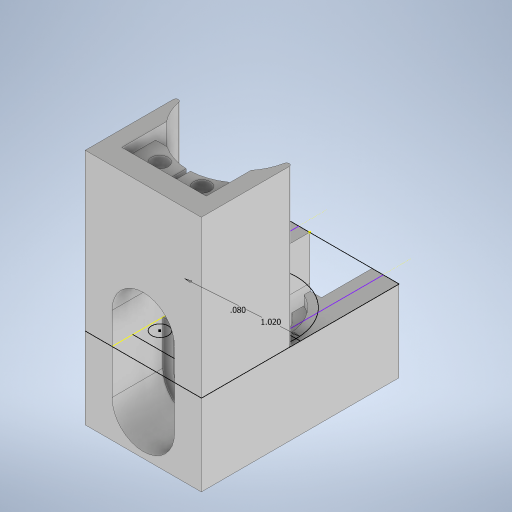
# Autodesk Inventor part: Ball Valve Mount 2
Saved by Autodesk Inventor 2024 (Build 280153000, 153)
## iProperties
Created: 2023-02-08
Part Number: Ball Valve Mount 2
Material: Generic
Document SubType Name: Modeling
Designer: tommy
Density: 1 g/cm^3
Appearance: Default
Author: tommy
Autodesk Inventor part; units mm, degrees
ref_plane "YZ Plane" through (0, 0, 0) normal (1, 0, 0) x (0, 1, 0)
ref_plane "XZ Plane" through (0, 0, 0) normal (0, 1, 0) x (-1, 0, 0)
ref_plane "XY Plane" through (0, 0, 0) normal (0, 0, 1) x (1, 0, 0)
sketch "Sketch1" plane through (0, 0, 0) normal (0, 1, 0) x (-1, 0, 0)
  circle A0 centre (0, 0) radius 8.636
  line L0 (7.5565, 23.7871) -> (-7.5565, 23.7871)
  line L1 (7.5565, -23.7871) -> (-7.5565, -23.7871)
  line L2 (7.5565, 23.7871) -> (7.5565, 8.2342)
  line L3 (7.5565, -8.2342) -> (7.5565, -23.7871)
  arc A1 (7.5565, -8.2342) -> (7.5565, 8.2342) centre (0, 0) ccw
  arc A2 (-7.5565, 8.2342) -> (-7.5565, -8.2342) centre (0, 0) ccw
  line L4 (-7.5565, -23.7871) -> (-7.5565, -8.2342)
  line L5 (-7.5565, 8.2342) -> (-7.5565, 23.7871)
  line L6 (-9.144, -8.9047) -> (-9.144, -23.7871)
  line L7 (9.144, -23.7871) -> (9.144, -8.9047)
  arc A3 (9.144, -8.9047) -> (9.144, 8.9047) centre (0, 0) ccw
  line L8 (9.144, 8.9047) -> (9.144, 23.7871)
  line L9 (-9.144, 23.7871) -> (-9.144, 8.9047)
  arc A4 (-9.144, 8.9047) -> (-9.144, -8.9047) centre (0, 0) ccw
  line L10 (7.5565, -23.7871) -> (9.144, -23.7871)
  line L11 (9.144, -23.7871) -> (-9.144, -23.7871)
  line L12 (-7.5565, 23.7871) -> (-9.144, 23.7871)
  line L13 (-9.144, 23.7871) -> (9.144, 23.7871)
  circle A5 centre (0, 0) radius 11.176
  line L14 (46.1577, 0) -> (-42.2099, 0)
  circle A6 centre (-19.5645, 19.9771) radius 2.0193
  circle A7 centre (0, 0) radius 2.921 construction
  circle A8 centre (0, 0) radius 6.604 construction
  line L15 (-6.3706, -6.3706) -> (-16.823, -4.7025) construction
  arc A9 (0, 23.3745) -> (-23.2624, -2.286) centre (0, 0) ccw construction
  line L16 (4.7025, 16.823) -> (6.3706, 6.3706) construction
  arc A10 (-20.8345, 0) -> (-16.823, -4.7025) centre (-16.0725, 0) ccw construction
  line L17 (-4.7025, -16.823) -> (-6.3706, -6.3706) construction
  arc A11 (-4.7025, -16.823) -> (0, -20.8345) centre (0, -16.0725) ccw construction
  arc A12 (4.7025, 16.823) -> (0, 20.8345) centre (0, 16.0725) ccw construction
  line L18 (6.3706, 6.3706) -> (16.823, 4.7025) construction
  arc A13 (20.8345, 0) -> (16.823, 4.7025) centre (16.0725, 0) ccw construction
  arc A14 (0, -20.8345) -> (20.8345, 0) centre (0, 0) ccw construction
  line L19 (2.286, -2.286) -> (-23.2624, -2.286) construction
  line L20 (-10.16, 30.48) -> (10.16, 30.48) construction
  circle A15 centre (-5.08, 34.544) radius 2.0193 construction
  line L21 (-13.97, 38.608) -> (13.97, 38.608) construction
  circle A16 centre (5.08, 34.544) radius 2.0193 construction
  line L22 (-0.508, 30.48) -> (-0.508, 38.608) construction
  line L23 (0.508, 30.48) -> (0.508, 38.608) construction
  line L24 (-10.16, -10.668) -> (-10.16, 30.48) construction
  line L25 (10.16, 9.906) -> (-10.16, 9.906) construction
  line L26 (13.97, 38.608) -> (13.97, -18.796) construction
  line L27 (-13.97, -18.796) -> (-13.97, 38.608) construction
  line L28 (10.16, 30.48) -> (10.16, -10.668) construction
  circle A17 centre (0, 0) radius 6.604 construction
  line L29 (10.16, -10.668) -> (-10.16, -10.668) construction
  circle A18 centre (5.08, -14.732) radius 2.0193 construction
  circle A19 centre (-5.08, -14.732) radius 2.0193 construction
  line L30 (-0.508, -18.796) -> (-0.508, -10.668) construction
  line L31 (0.508, -18.796) -> (0.508, -10.668) construction
  line L32 (-4.7025, -16.823) -> (-4.7191, -16.7188) construction
  line L33 (-4.7025, -16.823) -> (-4.7191, -16.7188) construction
  line L34 (13.97, -18.796) -> (-13.97, -18.796) construction
  arc A20 (0, 20.8345) -> (-20.8345, 0) centre (0, 0) ccw construction
  line L35 (0, 0) -> (0, 23.3745) construction
  line L36 (-23.3745, 0) -> (-23.3745, 23.7871)
  line L37 (-23.3745, 23.7871) -> (-9.144, 23.7871)
  line L38 (20.8345, 0) -> (20.8345, 23.7871)
  line L39 (20.8345, 23.7871) -> (9.144, 23.7871)
  line L40 (-23.3745, 0) -> (-23.3745, -18.796)
  line L41 (20.8345, 0) -> (20.8345, -18.796)
  arc A21 (-7.5565, 22.5203) -> (-23.3745, 4.2308) centre (0, 0) ccw
  arc A22 (7.5565, -19.8241) -> (20.8345, -4.0026) centre (0, 0) ccw
  arc A23 (20.8345, 1.9426) -> (17.0954, 5.0402) centre (16.0725, 0) ccw
  line L42 (17.0954, 5.0402) -> (11.748, 5.8959)
  circle A24 centre (0, 0) radius 12.7635 construction
  arc A25 (-20.4699, -2.667) -> (-16.883, -5.0787) centre (-16.0725, 0) ccw
  line L43 (-16.883, -5.0787) -> (-11.7468, -5.8984)
  line L44 (-20.4699, -2.667) -> (-23.3745, -2.667)
  arc A26 (-11.7468, -5.8984) -> (-7.5565, -10.7553) centre (0, 0) ccw
  arc A27 (11.748, 5.8959) -> (7.5565, 10.7553) centre (0, 0) ccw
  circle A28 centre (17.0245, 19.9771) radius 2.0193
  circle A29 centre (17.0245, -19.9771) radius 2.0193
  circle A30 centre (-17.0245, -17.4371) radius 2.0193
  line L45 (-9.144, -18.796) -> (-7.5565, -18.796)
  circle A31 centre (-19.5645, 19.9771) radius 2.286
  circle A32 centre (-17.0245, -17.4371) radius 2.286
  circle A33 centre (17.0245, -19.9771) radius 2.286
  circle A34 centre (17.0245, 19.9771) radius 2.286
  arc A35 (-9.144, 8.9047) -> (-9.144, -8.9047) centre (0, 0) ccw
  line L46 (-9.144, -8.9047) -> (-9.144, -18.796)
  line L47 (-23.3745, -18.796) -> (-23.3745, 23.7871)
  line L48 (-23.3745, 23.7871) -> (-9.144, 23.7871)
  line L49 (-9.144, 23.7871) -> (-9.144, 8.9047)
  line L50 (20.8345, -18.796) -> (20.8345, 23.7871)
  line L51 (20.8345, 23.7871) -> (9.144, 23.7871)
  line L52 (9.144, 23.7871) -> (9.144, 8.9047)
  line L53 (9.144, -18.796) -> (9.144, -8.9047)
  arc A36 (9.144, -8.9047) -> (9.144, 8.9047) centre (0, 0) ccw
  line L54 (9.144, -23.7871) -> (20.8345, -23.7871)
  line L55 (20.8345, -23.7871) -> (20.8345, -18.796)
  line L56 (-9.144, -23.7871) -> (-23.3745, -23.7871)
  line L57 (-23.3745, -23.7871) -> (-23.3745, -18.796)
  point P0 (-7.5565, -8.2342)
  point P1 (-7.5565, 8.2342)
  point P2 (-12.7635, 0)
  point P3 (-8.636, 0)
  point P4 (8.636, 0)
  point P5 (12.7635, 0)
  point P6 (-12.7635, 0)
  point P7 (0, 9.906)
  point P8 (-9.144, 21.9238)
  point P9 (9.8391, -18.796)
  point P10 (9.144, -19.1438)
  point P11 (-9.144, -9.4427)
  point P12 (-9.144, -9.4427)
  dimension "d12" = 18.161
  dimension "d0" = 17.272
  dimension "d6" = 15.113
  dimension "d7" = 1.5875
  dimension "d27" = 4.0386
  dimension "d31" = 5.842
  dimension "d32" = 13.208
  dimension "d38" = 41.148
  dimension "d39" = 20.32
  dimension "d40" = 4.0386
  dimension "d41" = 4.0386
  dimension "d49" = 13.208
  dimension "d55" = 3.81
  dimension "d56" = 3.81
  dimension "d57" = 19.5645
  dimension "d59" = 4.0386
  dimension "d60" = 4.0386
  dimension "d61" = 4.0386
  dimension "d62" = 3.81
  dimension "d64" = 6.35
  dimension "d66" = 3.81
  dimension "d67" = 3.81
  dimension "d68" = 4.572
  dimension "d69" = 4.572
  dimension "d70" = 4.572
  dimension "d71" = 4.572
  dimension "d90" = 3.81
  dimension "d91" = 6.35
  constraints: 114 end point, 44 point on circle, 35 centre point, 24 point on line, 16 perpendicular, 10 coincident, 5 parallel, 5 tangent, 4 horizontal, 4 vertical, 3 midpoint, 2 collinear, 1 concentric, 1 horizontal alignment, 15 other
  measures "d0" diameter of A0
  measures "d6" distance of L0.start L0.end
  measures "d7" distance between parallel lines of L4 L6
  measures "d27" diameter of A6
  measures "d31" diameter of A7
  measures "d32" diameter of A8
  measures "d38" distance of L28.start L28.end
  measures "d39" distance of L24.end L28.start
  measures "d40" diameter of A16
  measures "d41" diameter of A18
  measures "d49" diameter of A17
  measures "d55" distance from line of L36 A6.centre
  measures "d56" distance from line of L37 A6.centre
  measures "d57" distance from line of L35 A6.centre
  measures "d59" diameter of A28
  measures "d60" diameter of A29
  measures "d61" diameter of A30
  measures "d62" distance from line of L41 A29.centre
  measures "d64" distance from line of L40 A30.centre
  measures "d66" distance from line of L38 A28.centre
  measures "d67" distance from line of L39 A28.centre
  measures "d68" diameter of A31
  measures "d69" diameter of A32
  measures "d70" diameter of A33
  measures "d71" diameter of A34
  measures "d90" distance from line of L54 A29.centre
  measures "d91" distance from line of L56 A30.centre
extrude "Extrusion1" add sketch "Sketch1" along normal blind 18.796 contours A0 L14 A2 A5 A1 | A1 L2 A27 L8 A3 L14 | L14 A4 L9 A21 L5 A2 | A5 L5 L0 L2 | L2 L13 L8 A27 | A21 L9 L12 L5 picked at (-5.9238, 8.392)
extrude "Extrusion2" cut sketch "Sketch1" along normal blind 2.286 contours L14 A1 A5 A2 A0 | A0 L14 A2 A5 A1
sketch "Sketch2" plane through (-9.144, 0, 23.7871) normal (0, 0, 1) x (1, 0, 0)
  line L0 (9.144, 0) -> (9.144, 18.161)
  line L1 (9.144, 18.161) -> (9.144, 10.6426)
  circle A0 centre (9.144, 10.6426) radius 7.5184
  line L2 (16.6624, 10.6426) -> (16.6624, -7.5184)
  line L3 (20.32, 0) -> (-2.032, 0) projected
  line L4 (1.6256, 10.6426) -> (1.6256, -7.5184)
  line L5 (1.6256, 0) -> (16.6624, 0)
  circle A1 centre (9.144, 10.6426) radius 4.826
  line L6 (4.318, 10.6426) -> (4.318, 0)
  line L7 (13.97, 10.6426) -> (13.97, 0)
  line L8 (18.288, 0) -> (0, 0) projected
  circle A2 centre (9.144, -7.5184) radius 7.5184
  line L9 (1.6256, 10.6426) -> (16.6624, 10.6426)
  point P0 (4.318, 0)
  point P1 (4.318, 5.7651)
  point P2 (13.97, 5.7651)
  point P3 (9.144, 7.5184)
  dimension "d12" = 18.161
  dimension "d13" = 7.5184
  dimension "d17" = 9.652
  constraints: 16 end point, 8 point on line, 7 point on circle, 3 centre point, 3 perpendicular, 2 coincident, 2 vertical, 1 horizontal, 1 parallel
  measures "d12" distance of L0.start L0.end
  measures "d13" distance of L0.end L1.end
  measures "d17" diameter of A1
extrude "Extrusion3" cut sketch "Sketch2" against normal blind 254 contours L3 L6 A0 L0 | L0 A0 L7 L3 | A0 L6 A1 L0 | L0 A1 L7 A0 | A1 L9 L0 | L0 L9 A1 | L9 A1 L0 | L0 A1 L9
extrude "Extrusion4" cut sketch "Sketch2" against normal blind 12.2174 contours L7 A0 L2 L3 | L3 L4 A0 L6 | A0 L9 L6 | L7 L9 A0 | L9 A0 L0 A1 | A1 L0 A0 L9
mirror "Mirror3" about plane through (12.7635, 0, 0) normal (0, 0, -1)
sketch "Sketch5" plane through (0, 18.796, 0) normal (0, 1, 0) x (1, 0, 0)
  arc A0 (-9.144, 8.9047) -> (-9.144, -8.9047) centre (0, 0) ccw projected
  line L0 (-9.144, 8.9047) -> (-9.144, 23.7871) projected
  line L1 (-12.7635, 0) -> (12.7635, 0)
  line L2 (13.97, -23.7871) -> (-13.97, -23.7871)
  line L3 (-13.97, -23.7871) -> (-13.97, 23.7871)
  line L4 (-13.97, 23.7871) -> (13.97, 23.7871)
  line L5 (13.97, 23.7871) -> (13.97, -23.7871)
  arc A1 (-4.826, 10.0803) -> (-4.826, -10.0803) centre (0, 0) ccw projected
  line L6 (13.97, -23.7871) -> (-13.97, 23.7871) construction
  line L7 (-13.97, -23.7871) -> (13.97, 23.7871) construction
  line L8 (9.144, 23.7871) -> (9.144, 8.9047) projected
  arc A2 (9.144, -8.9047) -> (9.144, 8.9047) centre (0, 0) ccw projected
  line L9 (9.144, -23.7871) -> (9.144, -8.9047) projected
  line L10 (-9.144, -8.9047) -> (-9.144, -23.7871) projected
  circle A3 centre (0, 0) radius 8.636 projected
  arc A4 (9.144, -8.9047) -> (9.144, 8.9047) centre (0, 0) ccw projected
  line L11 (9.144, 23.7871) -> (9.144, 8.9047) projected
  line L12 (-9.144, 23.7871) -> (9.144, 23.7871) projected
  line L13 (-9.144, 8.9047) -> (-9.144, 23.7871) projected
  arc A5 (-9.144, 8.9047) -> (-9.144, -8.9047) centre (0, 0) ccw projected
  line L14 (-9.144, -8.9047) -> (-9.144, -23.7871) projected
  line L15 (-9.144, -23.7871) -> (9.144, -23.7871) projected
  line L16 (9.144, -23.7871) -> (9.144, -8.9047) projected
  point P0 (13.97, 0)
  point P1 (-13.97, 0)
  dimension "d120" = 27.94
  dimension "d121" = 0
  constraints: 14 end point, 2 midpoint, 2 parallel, 2 point on circle, 1 horizontal, 1 perpendicular
  measures "d120" distance between parallel lines of L5 L3
  measures "d121" distance between parallel lines of L12 L4
extrude "Extrusion9" add sketch "Sketch5" against normal up to surface (18.796 mm away) contours A0 L10 L2 L3 L4 L0 | L4 L5 L2 L9 A2 L8
extrude "Extrusion10" add sketch "Sketch5" along normal blind 0.7937
sketch "Sketch6" plane through (0, 0, 0) normal (0, -1, 0) x (1, 0, 0)
  circle A0 centre (-5.08, -14.732) radius 2.0193 construction
  circle A1 centre (5.08, -14.732) radius 2.0193 construction
  line L0 (10.16, -10.668) -> (10.16, 30.48) construction
  line L1 (-10.16, 30.48) -> (-10.16, -10.668) construction
  circle A2 centre (-5.08, -14.732) radius 2.0193
  circle A3 centre (5.08, -14.732) radius 2.0193
  line L2 (-13.97, -18.796) -> (13.97, -18.796) construction
  line L3 (-10.16, -10.668) -> (10.16, -10.668) construction
  line L4 (-7.5565, -8.2342) -> (-7.5565, -23.7871) projected
  line L5 (7.5565, -23.7871) -> (7.5565, -8.2342) projected
  line L6 (7.5184, 23.7871) -> (13.97, 23.7871) projected
  line L7 (13.97, 23.7871) -> (-13.97, 23.7871) projected
  line L8 (10.16, -18.796) -> (-10.16, -18.796)
  line L9 (10.16, -18.796) -> (10.16, 23.7871)
  line L10 (-10.16, -18.796) -> (-10.16, 23.7871)
  line L11 (10.16, 23.7871) -> (13.97, 23.7871)
  line L12 (13.97, -23.7871) -> (13.97, 23.7871) projected
  line L13 (13.97, 23.7871) -> (13.97, -23.7871)
  line L14 (13.97, -23.7871) -> (-13.97, -23.7871)
  line L15 (-13.97, -23.7871) -> (-13.97, 23.7871)
  line L16 (-13.97, 23.7871) -> (13.97, 23.7871)
  line L17 (-13.97, 0) -> (13.97, 0)
  line L18 (-12.7635, -2.032) -> (12.7635, -2.032)
  circle A4 centre (0, 0) radius 12.954
  point P0 (-7.5184, 23.7871)
  point P1 (-7.5184, 23.7871)
  point P2 (13.97, 0)
  point P3 (-12.7635, -2.2134)
  point P4 (12.7635, -2.2134)
  point P5 (12.954, 0)
  point P6 (-12.954, 0)
  dimension "d105" = 2.032
  dimension "d106" = 25.908
  constraints: 20 end point, 6 point on line, 3 centre point, 3 coincident, 2 concentric, 2 horizontal, 2 midpoint, 2 perpendicular, 1 parallel, 1 vertical
  measures "d105" distance between parallel lines of L17 L18
  measures "d106" diameter of A4
extrude "Extrusion11" add sketch "Sketch6" along normal blind 35.1282 contours A4 L5 L8 L4 | L4 L8 L10 A4 | L8 L5 L14 L4 | L4 L14 L15 L17 A4 L10 L8 | A4 L9 L8 L5 | L8 L9 A4 L17 L12 L14 L5
sketch "Sketch7" plane through (0, -35.1282, 0) normal (0, -1, 0) x (1, 0, 0)
  arc A0 (-5.8265, -11.5697) -> (5.8265, -11.5697) centre (0, 0) ccw projected
  line L0 (0, -12.954) -> (0, -23.7871)
  line L1 (-13.97, -23.7871) -> (13.97, -23.7871) projected
  line L2 (0.508, -12.944) -> (0.508, -23.7871)
  line L3 (-0.508, -12.944) -> (-0.508, -23.7871)
  line L4 (-13.97, -18.796) -> (13.97, -18.796) construction
  arc A1 (-12.954, 0) -> (12.954, 0) centre (0, 0) ccw projected
  arc A2 (12.7635, -3.381) -> (12.5138, -3.3482) centre (12.6365, -3.381) ccw projected
  arc A3 (-12.5138, -3.3482) -> (-12.7635, -3.381) centre (-12.6365, -3.381) ccw projected
  line L5 (-13.97, 0) -> (-13.97, -23.7871) projected
  line L6 (13.97, -23.7871) -> (13.97, 0) projected
  line L7 (10.16, -8.0362) -> (10.16, -18.796)
  line L8 (10.16, -18.796) -> (-10.16, -18.796)
  line L9 (-10.16, -18.796) -> (-10.16, -8.0362)
  line L10 (-10.16, -10.668) -> (10.16, -10.668) construction
  line L11 (-10.16, -10.668) -> (10.16, -10.668)
  line L12 (-10.16, -10.668) -> (10.16, -10.668)
  line L13 (10.16, -10.668) -> (10.16, -8.0362)
  line L14 (10.16, -8.0362) -> (-10.16, -8.0362)
  line L15 (-10.16, -8.0362) -> (-10.16, -10.668)
  point P0 (0.508, -12.954)
  point P1 (-0.508, -12.954)
  point P2 (-7.3485, -10.668)
  point P3 (7.3485, -10.668)
  point P4 (13.97, 0)
  point P5 (0.508, -18.796)
  point P6 (-0.508, -18.796)
  dimension "d108" = 0.508
  constraints: 22 end point, 4 point on line, 3 parallel, 3 point on circle, 2 symmetric about line, 1 collinear, 1 horizontal, 1 midpoint, 1 perpendicular, 5 other
  measures "d108" distance between parallel lines of L0 L2
extrude "Extrusion12" cut sketch "Sketch7" against normal blind 2.54 contours A0 L0 L8 L3 | A0 L2 L8 L0
extrude "Extrusion13" cut sketch "Sketch2" against normal blind 53.34 contours A2 L4 L3 | L3 L2 A2 | A2
fillet "Fillet3" [suppressed]
extrude "Extrusion16" cut sketch "Sketch7" against normal blind 9.652 contours L11 L9 A1 | A1 L7 L11
fillet "Fillet4" radius 0.635 2 edges at (-13.97, -17.5641, 0) (-12.954, -17.5641, 0)
fillet "Fillet5" radius 0.635 2 edges at (13.97, -17.5641, 0) (12.954, -17.5641, 0)
sketch "Sketch8" plane through (0, -35.1282, 0) normal (0, -1, 0) x (1, 0, 0)
  arc A0 (13.97, -2.6151) -> (12.7119, -2.4929) centre (13.335, -2.6151) ccw projected
  arc A1 (-12.954, 0) -> (12.954, 0) centre (0, 0) ccw projected
  line L0 (13.97, -23.7871) -> (13.97, 0) projected
  line L1 (-13.97, -23.7871) -> (13.97, -23.7871) projected
  line L2 (-13.97, 0) -> (-13.97, -23.7871) projected
  arc A2 (-12.7119, -2.4929) -> (-13.97, -2.6151) centre (-13.335, -2.6151) ccw projected
  line L3 (-10.16, -18.796) -> (-10.16, -8.0362) projected
  line L4 (10.16, -18.796) -> (-10.16, -18.796) projected
  line L5 (10.16, -8.0362) -> (10.16, -18.796) projected
extrude "Extrusion17" add sketch "Sketch8" along normal blind 2.54 contours L0 L1 L2 A2 A1 L3 L4 L5 A0
body "Solid1"
